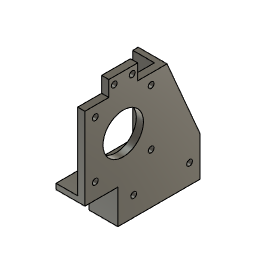
MotorMounts (Autodesk Fusion 360 design; units mm, degrees)
Autodesk Fusion 360 part; units mm, degrees
sketch "motor_mount" plane through (0, 0, 0) normal (1, 0, 0) x (0, 1, 0)
  circle A0 centre (0, 0) radius 11.25
  line L0 (15.5, 15.5) -> (-15.5, 15.5) construction
  line L1 (-15.5, 15.5) -> (-15.5, -15.5) construction
  line L2 (-15.5, -15.5) -> (15.5, -15.5) construction
  line L3 (15.5, -15.5) -> (15.5, 15.5) construction
  line L4 (15.5, 15.5) -> (-15.5, -15.5) construction
  line L5 (-15.5, 15.5) -> (15.5, -15.5) construction
  line L6 (21.3, 21.3) -> (-21.3, 21.3)
  line L7 (-21.3, 21.3) -> (-21.3, -21.3)
  line L8 (-21.3, -21.3) -> (21.3, -21.3)
  line L9 (21.3, -21.3) -> (21.3, 21.3)
  line L10 (21.3, 21.3) -> (-21.3, -21.3) construction
  line L11 (-21.3, 21.3) -> (21.3, -21.3) construction
  line L12 (-21.3, -21.3) -> (21.3, -21.3)
  line L13 (-21.3, -21.3) -> (21.3, -21.3)
  line L14 (21.3, -24.3) -> (-21.3, -24.3)
  line L15 (-21.3, -24.3) -> (-21.3, -21.3)
  circle A1 centre (-15.5, 15.5) radius 1.6
  circle A2 centre (15.5, 15.5) radius 1.6
  circle A3 centre (-15.5, -15.5) radius 1.6
  circle A4 centre (15.5, -15.5) radius 1.6
  circle A5 centre (36.8, -32.5) radius 1.6
  circle A6 centre (5.8, -32.5) radius 1.6
  line L16 (5.8, -32.5) -> (36.8, -32.5) construction
  line L17 (0, -24.3) -> (-3, -24.3)
  line L18 (-3, -24.3) -> (-3, -43.3)
  line L19 (-3, -43.3) -> (0, -43.3)
  line L20 (0, -43.3) -> (0, -24.3)
  line L21 (0, -43.3) -> (42.6, -43.3)
  line L22 (42.6, -43.3) -> (42.6, -24.3)
  line L23 (42.6, -24.3) -> (21.3, -24.3)
  line L24 (21.3, -21.3) -> (42.6, -21.3)
  line L25 (42.6, -21.3) -> (42.6, -24.3)
  line L26 (21.3, 21.3) -> (24.3, 21.3)
  line L27 (24.3, 21.3) -> (24.3, -21.3)
  line L28 (24.3, -21.3) -> (21.3, -21.3)
  line L29 (21.3, -21.3) -> (21.3, 21.3)
  line L30 (24.3, 21.3) -> (42.6, -21.3)
  line L31 (0, 21.3) -> (-8, 21.3)
  line L32 (-8, 21.3) -> (8, 21.3)
  line L33 (8, 21.3) -> (8, 29.9)
  line L34 (8, 29.9) -> (-8, 29.9)
  line L35 (-8, 29.9) -> (-8, 21.3)
  circle A7 centre (-5, 26) radius 1.6
  circle A8 centre (5, 26) radius 1.6
  dimension "d1" = 22.5
  dimension "d2" = 31
  dimension "d3" = 31
  dimension "d5" = 42.6
  dimension "d6" = 42.6
  dimension "d8" = 3
  dimension "d9" = 3.2
  dimension "d10" = 3.2
  dimension "d11" = 3.2
  dimension "d12" = 3.2
  dimension "d13" = 3.2
  dimension "d14" = 3.2
  dimension "d267" = 31
  dimension "d268" = 3
  dimension "d269" = 19
  dimension "d270" = 42.6
  dimension "d271" = 3
  dimension "d286" = 8
  dimension "d287" = 16
  dimension "d288" = 8.6
  dimension "d323" = 3.2
  dimension "d324" = 3.2
  constraint coincident A0.centre origin
  constraint horizontal L0
  constraint perpendicular L0 L1
  constraint parallel L0 L2
  constraint parallel L1 L3
  constraint coincident L4 A0.centre
  constraint coincident L5 A0.centre
  constraint horizontal L6
  constraint perpendicular L6 L7
  constraint parallel L6 L8
  constraint parallel L7 L9
  constraint coincident L10 A0.centre
  constraint coincident L11 A0.centre
  constraint horizontal L12
  constraint horizontal L13
  constraint horizontal L14
  constraint vertical L15
  constraint coincident L0.end L1.start
  constraint coincident L0.start L3.end
  constraint coincident L1.end L2.start
  constraint coincident L2.end L3.start
  constraint coincident A6.centre L16.start
  constraint coincident A5.centre L16.end
  constraint horizontal L16
  constraint horizontal L17
  constraint vertical L18
  constraint horizontal L19
  constraint vertical L20
  constraint midpoint L14 L17.start
  constraint perpendicular L20 L21
  constraint perpendicular L14 L22
  constraint perpendicular L22 L23
  constraint perpendicular L9 L24
  constraint perpendicular L23 L25
  constraint horizontal L26
  constraint vertical L27
  constraint horizontal L28
  constraint vertical L29
  constraint coincident L24 L27.end
  constraint midpoint L6 L31.start
  constraint parallel L6 L31
  constraint horizontal L32
  constraint vertical L33
  constraint horizontal L34
  constraint vertical L35
  measures "d1" diameter of A0
  measures "d2" distance of L1.end L2.end
  measures "d3" distance of L0.end L1.end
  measures "d5" distance of L6.end L7.end
  measures "d6" distance of L7.end L8.end
  measures "d8" distance of L7.end L14.end
  measures "d9" diameter of A1
  measures "d10" diameter of A2
  measures "d11" diameter of A3
  measures "d12" diameter of A4
  measures "d13" diameter of A5
  measures "d14" diameter of A6
  measures "d267" distance of A6.centre A5.centre
  measures "d268" distance of L17.start L17.end
  measures "d269" distance of L17.start L19.end
  measures "d270" distance of L19.end L21.end
  measures "d271" distance of L6.start L26.end
  measures "d286" distance of L31.start L31.end
  measures "d287" distance of L31.end L32.end
  measures "d288" distance of L31.end L34.end
  measures "d323" diameter of A8
  measures "d324" diameter of A7
extrude "Extrude1" add sketch "motor_mount" along normal blind 4 makes body 1
extrude "Extrude2" add sketch "motor_mount" against normal blind 12 contours L9 L24 L26 L27 L28 L29 | L8 L12 L13 L14 L15 L17 L23 L24 L25 L28 | L14 L17 L18 L19 L20 bodies 1
mirror "Mirror1" about plane through (0, 0, 0) normal (0, 1, 0) of bodies 1 makes body 2
hidden bodies 2
equation "pen_min_diam = 8 mm"
equation "pen_max_diam = 13 mm"
equation "pen_holder_diam = 17 mm"
equation "pen_shaft_diam = 23 mm"
equation "pen_sled_diam = 50 mm"
equation "pen_bearing_tolerance = 0.7 mm"
equation "pen_support_diam = 36 mm"
equation "pen_shaft_tolerance = 0.8 mm"
equation "sled_thickness = 4 mm"
equation "bearing_offset_ring_thickness = 0.5 mm"
equation "assembly_tolerance = 0.2 mm"
equation "bearing_1_plane = sled_thickness + bearing_offset_ring_thickness + assembly_tolerance"
equation "bearing_thickness = 3.6 mm"
equation "bearing_2_plane = bearing_1_plane + bearing_thickness + assembly_tolerance"
equation "bearing_cap_plane = bearing_2_plane + bearing_thickness + bearing_offset_ring_thickness + assembly_tolerance"
equation "bearing_cap_threaded_thickness = 4 mm"
equation "bearing_cap_supported_thickness = 4 mm"
equation "bearing_cap_height = 20 mm"
named bodies: "motor_mount_left", "motor_mount_right"
